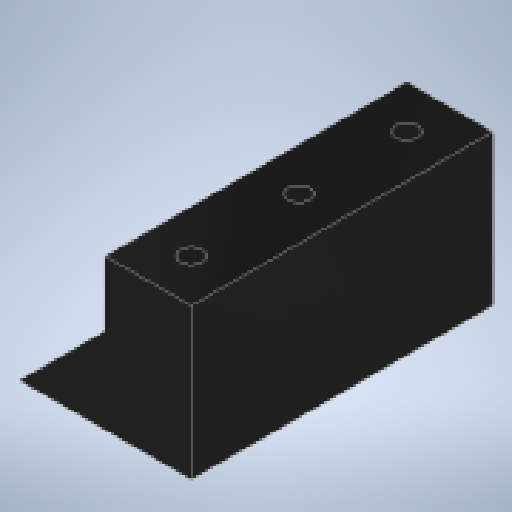
# Autodesk Inventor part: Magazine_Mount_Plate_Spacer
Saved by Autodesk Inventor 2025.1 (Build 291241020, 241B)
## iProperties
Created: 2024-11-14
Part Number: Magazine_Mount_Plate_Spacer
Material: PC/ABS Plastic
Document SubType Name: Modeling
Designer: leon-
Density: 1.1 g/cm^3
Appearance: Smooth - Black
Author: leon-
Autodesk Inventor part; units mm, degrees
ref_plane "YZ Plane" through (0, 0, 0) normal (1, 0, 0) x (0, 1, 0)
ref_plane "XZ Plane" through (0, 0, 0) normal (0, 1, 0) x (-1, 0, 0)
ref_plane "XY Plane" through (0, 0, 0) normal (0, 0, 1) x (1, 0, 0)
sketch "Sketch1" plane through (0, 0, 0) normal (0, 1, 0) x (-1, 0, 0)
  line L0 (0, 0) -> (20, 0)
  line L1 (20, 0) -> (20, -70)
  line L2 (20, -70) -> (0, -70)
  line L3 (0, -70) -> (0, 0)
  dimension "d0" = 70
  dimension "d1" = 20
  constraints: 8 end point, 2 parallel, 1 horizontal, 1 perpendicular
  measures "d0" distance of L0.end L1.end
  measures "d1" distance of L1.end L2.end
extrude "Extrusion1" add sketch "Sketch1" along normal blind 35
sketch "Sketch2" plane through (0, 35, 0) normal (0, 1, 0) x (1, 0, 0)
  line L0 (-20, 70) -> (-20, 0) projected
  line L1 (0, 70) -> (-20, 70) projected
  point P0 (0, 0)
  point P1 (-10, 60)
  point P2 (-20, 35)
  point P3 (-10, 70)
  point P4 (-10, 35)
  point P5 (-10, 10)
  dimension "d5" = 10
  dimension "d6" = 10
  dimension "d14" = 25
  dimension "d15" = 25
  constraints: 2 midpoint, 2 vertical alignment
  measures "d5" distance from line of L0 point (-10, 60)
  measures "d6" distance of point (-10, 70) point (-10, 60)
  measures "d14" distance of point (-10, 35) point (-10, 10)
  measures "d15" distance of point (-10, 60) point (-10, 35)
hole "Hole1" at (-10, 35, -60) at (-10, 35, -35) at (-10, 35, -10) direction (0, -1, 0) diameter 5 end through all
sketch "Sketch3" plane through (0, 0, -70) normal (0, 0, -1) x (-1, 0, 0)
  line L0 (0, 0) -> (20, 0) projected
  line L1 (20, 0) -> (20, 20)
  line L2 (20, 0) -> (20, 35) projected
  line L3 (20, 20) -> (40, 0)
  line L4 (40, 0) -> (20, 0)
  dimension "d16" = 20
  dimension "d17" = 45
  constraints: 6 end point, 1 perpendicular, 1 point on line
  measures "d16" distance of L0.end L1.end
  measures "d17" angle of L1 L3
extrude "Extrusion2" add sketch "Sketch3" against normal up to surface (70 mm away)
body "Solid1"
